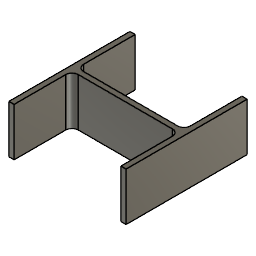
H-244×252×11×11 (Autodesk Fusion 360 design; units mm, degrees)
Autodesk Fusion 360 part; units mm, degrees
sketch "スケッチ1" plane through (0, 0, 0) normal (0, 0, 1) x (1, 0, 0)
  line L0 (0, 126) -> (0, -126)
  line L1 (244, -126) -> (244, 126)
  line L2 (233, -18.5) -> (233, -126)
  line L3 (11, -126) -> (11, -18.5)
  line L4 (0, -126) -> (11, -126)
  line L5 (233, -126) -> (244, -126)
  line L6 (220, 5.5) -> (24, 5.5)
  line L7 (24, -5.5) -> (220, -5.5)
  line L8 (11, 18.5) -> (11, 126)
  line L9 (11, 126) -> (0, 126)
  line L10 (233, 126) -> (233, 18.5)
  line L11 (244, 126) -> (233, 126)
  arc A0 (24, -5.5) -> (11, -18.5) centre (24, -18.5) ccw
  arc A1 (11, 18.5) -> (24, 5.5) centre (24, 18.5) ccw
  arc A2 (220, 5.5) -> (233, 18.5) centre (220, 18.5) ccw
  arc A3 (233, -18.5) -> (220, -5.5) centre (220, -18.5) ccw
extrude "押し出し1" add sketch "スケッチ1" along normal blind 100
